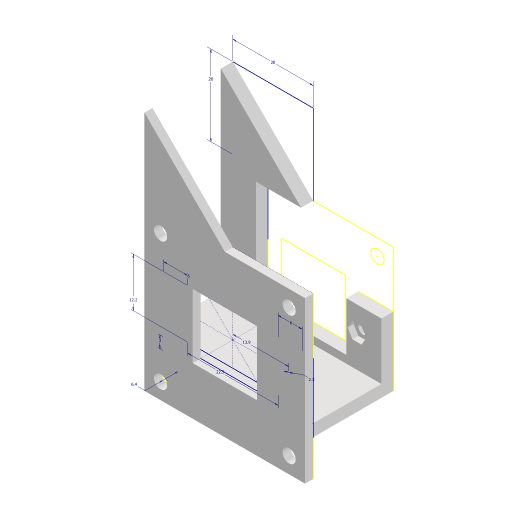
# Autodesk Inventor part: SG90_holder_1205
Saved by Autodesk Inventor 2024 (Build 280153000, 153)
## iProperties
Created: 2023-02-14
Part Number: SG90_holder_1205
Material: 一般
Document SubType Name: Modeling
Designer: USER
Density: 1 g/cm^3
Appearance: 預設
Author: USER
Autodesk Inventor part; units mm, degrees
ref_plane "YZ Plane" through (0, 0, 0) normal (1, 0, 0) x (0, 1, 0)
ref_plane "XZ Plane" through (0, 0, 0) normal (0, 1, 0) x (-1, 0, 0)
ref_plane "XY Plane" through (0, 0, 0) normal (0, 0, 1) x (1, 0, 0)
sketch "草圖11" plane through (0, 0, 0) normal (0, 0, 1) x (1, 0, 0)
  line L0 (0, 0) -> (22.5, 0)
  line L1 (22.5, 0) -> (22.5, -12.2)
  line L2 (22.5, -12.2) -> (0, -12.2)
  line L3 (0, -12.2) -> (0, 0)
  line L4 (-6, -18.2) -> (28.5, -18.2)
  line L5 (28.5, -18.2) -> (28.5, 6)
  line L6 (28.5, 6) -> (-6, 6)
  line L7 (-6, 6) -> (-6, -18.2)
  circle A0 centre (-2.65, -6.1) radius 1.15
  line L8 (0, -6.1) -> (22.5, -6.1) construction
  line L9 (11.25, 0) -> (11.25, -12.2) construction
  circle A1 centre (25.15, -6.1) radius 1.15
  line L10 (-6, 0) -> (0, 0) construction
  line L11 (22.5, 0) -> (28.5, 0) construction
  line L12 (-6, 0) -> (0, 0)
  line L13 (22.5, 0) -> (28.5, 0)
  line L14 (22.5, 0) -> (22.5, 6)
  line L15 (0, 0) -> (0, 6)
  dimension "d52" = 22.5
  dimension "d53" = 12.2
  dimension "d55" = 2.3
  dimension "d56" = 13.9
  dimension "d110" = 6
  constraints: 32 end point, 6 point on line, 5 equal length, 5 perpendicular, 4 midpoint, 2 centre point, 2 horizontal, 1 symmetric about line, 4 other
  measures "d52" distance of L1.end L2.end
  measures "d53" distance of L0.end L1.end
  measures "d55" diameter of A0
  measures "d56" distance from line of L9 A0.centre
  measures "d110" distance between parallel lines of L4 L2
extrude "擠出11" [suppressed]
sketch "草圖20" plane through (0, 0, 2) normal (0, 0, 1) x (1, 0, 0)
  line L0 (28.5, 0) -> (22.5, 0) projected
  line L1 (22.5, 0) -> (22.5, -12.2) projected
  line L2 (22.5, -12.2) -> (0, -12.2) projected
  line L3 (0, -12.2) -> (0, 0) projected
  line L4 (0, 0) -> (-6, 0) projected
  line L5 (-6, 0) -> (-6, -18.2) projected
  line L6 (-6, -18.2) -> (28.5, -18.2) projected
  line L7 (28.5, -18.2) -> (28.5, 0) projected
  circle A0 centre (-2.65, -6.1) radius 1.15 projected
  circle A1 centre (25.15, -6.1) radius 1.15 projected
  line L8 (-6, 0) -> (-4, 0)
  line L9 (-4, 0) -> (-4, -18.2)
  line L10 (-4, -18.2) -> (-6, -18.2)
  line L11 (-6, -18.2) -> (-6, 0)
  line L12 (-6, -18.2) -> (28.5, -18.2)
  line L13 (28.5, -18.2) -> (28.5, -16.2)
  line L14 (28.5, -16.2) -> (-6, -16.2)
  line L15 (-6, -16.2) -> (-6, -18.2)
  line L16 (-6, -18.2) -> (28.5, -18.2) projected
  point P0 (-4, -16.2)
  dimension "d97" = 2
  dimension "d98" = 2
  constraints: 16 end point, 4 parallel, 3 point on line, 2 horizontal, 2 perpendicular, 1 collinear
  measures "d97" distance between parallel lines of L5 L9
  measures "d98" distance between parallel lines of L6 L14
extrude "擠出17" [suppressed]
sketch "草圖21" plane through (0, 0, 22) normal (0, 0, 1) x (1, 0, 0)
  line L0 (-8.75, -26.1) -> (31.25, -26.1)
  line L1 (31.25, -26.1) -> (31.25, 13.9)
  line L2 (31.25, 13.9) -> (-8.75, 13.9)
  line L3 (-8.75, 13.9) -> (-8.75, -26.1)
  circle A0 centre (-2.65, -6.1) radius 1.15 projected
  line L4 (-8.75, -6.1) -> (31.25, -6.1) construction
  line L5 (11.25, -26.1) -> (11.25, 13.9) construction
  line L6 (28.5, -16.2) -> (-4, -16.2) construction
  line L7 (-4, -16.2) -> (-4, 0) construction
  line L8 (-4, 0) -> (-6, 0) construction
  line L9 (-6, 0) -> (-6, -18.2) construction
  line L10 (-6, -18.2) -> (28.5, -18.2) construction
  line L11 (28.5, -18.2) -> (28.5, -16.2) construction
  line L12 (-6, -18.2) -> (28.5, -18.2) construction
  line L13 (11.25, -18.2) -> (11.25, -16.2) construction
  line L14 (28.5, -16.2) -> (-4, -16.2) construction
  line L15 (1.25, 3.9) -> (21.25, 3.9)
  line L16 (21.25, 3.9) -> (21.25, -16.1)
  line L17 (21.25, -16.1) -> (1.25, -16.1)
  line L18 (1.25, -16.1) -> (1.25, 3.9)
  circle A1 centre (-4.75, -22.1) radius 3 construction
  circle A2 centre (-4.75, -22.1) radius 1.65
  circle A3 centre (-4.75, 9.9) radius 1.65
  circle A4 centre (27.25, -22.1) radius 1.65
  circle A5 centre (27.25, 9.9) radius 1.65
  line L19 (1.25, 3.9) -> (1.25, 13.9)
  line L20 (21.25, -16.1) -> (31.25, -16.1)
  point P0 (0, 0)
  dimension "d101" = 40
  dimension "d102" = 40
  dimension "d103" = 10
  dimension "d104" = 3.3
  dimension "d105" = 6
  dimension "d106" = 16
  dimension "d107" = 16
  constraints: 26 end point, 5 centre point, 5 midpoint, 5 perpendicular, 4 parallel, 4 point on line, 3 symmetric about line, 1 coincident, 1 collinear, 1 horizontal, 6 other
  measures "d101" distance of L1.end L2.end
  measures "d102" distance of L2.end L0.start
  measures "d103" distance between parallel lines of L2 L15
  measures "d104" diameter of A2
  measures "d105" diameter of A1
  measures "d106" distance from line of L4 A1.centre
  measures "d107" distance from line of L5 A1.centre
extrude "擠出18" [suppressed]
sketch "草圖22" plane through (0, 0, 0) normal (0, 0, 1) x (1, 0, 0)
  line L0 (-20, 20) -> (20, 20)
  line L1 (20, 20) -> (20, -20)
  line L2 (20, -20) -> (-20, -20)
  line L3 (-20, -20) -> (-20, 20)
  line L4 (0, -12.2) -> (0, 0) projected
  line L5 (-20, 20) -> (20, -20) construction
  line L6 (20, 20) -> (-20, -20) construction
  line L7 (-16, 16) -> (16, 16) construction
  line L8 (16, 16) -> (16, -16) construction
  line L9 (16, -16) -> (-16, -16) construction
  line L10 (-16, -16) -> (-16, 16) construction
  line L11 (-16, 16) -> (16, -16) construction
  line L12 (16, 16) -> (-16, -16) construction
  circle A0 centre (-16, 16) radius 1.65
  line L13 (20, 20) -> (-8, 20)
  line L14 (-8, 20) -> (-8, -8)
  line L15 (-8, -8) -> (20, -8)
  line L16 (20, -8) -> (20, 20)
  circle A1 centre (-16, -16) radius 1.65
  circle A2 centre (16, 16) radius 1.65
  circle A3 centre (16, -16) radius 1.65
  line L17 (-8, 8) -> (8, 8)
  line L18 (8, 8) -> (8, -8)
  line L19 (8, -8) -> (-8, -8)
  line L20 (-8, -8) -> (-8, 8)
  point P0 (20, -8)
  dimension "d118" = 40
  dimension "d119" = 16
  dimension "d120" = 3.3
  dimension "d121" = 12
  dimension "d124" = 32
  dimension "d127" = 32
  constraints: 40 end point, 8 parallel, 5 perpendicular, 4 centre point, 4 horizontal, 4 midpoint, 2 point on line, 1 coincident, 1 collinear, 1 vertical, 9 other
  measures "d118" distance of L0.start L0.end
  measures "d119" distance from line of L4.end L8
  measures "d120" diameter of A0
  measures "d121" distance between parallel lines of L2 L15
  measures "d124" distance of A0.centre A1.centre
  measures "d127" distance of A0.centre A2.centre
extrude "擠出19" add sketch "草圖22" along normal blind 2 contours L0 L14 L15 L1 L2 L3 | L0 L1 L15 L18 L17 L14
sketch "草圖23" plane through (0, 0, 0) normal (0, 0, -1) x (-1, 0, 0)
  line L0 (-11.25, 6.1) -> (11.25, 6.1)
  line L1 (11.25, 6.1) -> (11.25, -6.1)
  line L2 (11.25, -6.1) -> (-11.25, -6.1)
  line L3 (-11.25, -6.1) -> (-11.25, 6.1)
  circle A0 centre (-13.9, 0) radius 1.15
  line L4 (-11.25, 0) -> (11.25, 0) construction
  line L5 (0, 6.1) -> (0, -6.1) construction
  circle A1 centre (13.9, 0) radius 1.15
  line L6 (20, -20) -> (-20, -20) projected
  circle A2 centre (16, -16) radius 1.65 projected
  line L7 (20, 20) -> (-20, 20) construction
  line L8 (-20, 20) -> (-20, -20) construction
  line L9 (-20, -20) -> (20, -20) construction
  line L10 (20, -20) -> (20, 20) construction
  line L11 (20, 20) -> (-20, -20) construction
  line L12 (-20, 20) -> (20, -20) construction
  line L13 (17.25, 6.1) -> (-17.25, 6.1)
  line L14 (-17.25, 6.1) -> (-17.25, -11)
  line L15 (-17.25, -11) -> (17.25, -11)
  line L16 (17.25, -11) -> (17.25, 6.1)
  circle A3 centre (16, -16) radius 3.2 construction
  line L17 (17.25, -8) -> (-17.25, -8)
  line L18 (-8, -8) -> (8, -8) construction
  line L19 (20, 6.1) -> (17.25, 6.1)
  line L20 (17.25, -8) -> (20, -8)
  line L21 (17.25, -11) -> (20, -11)
  line L22 (20, 6.1) -> (20, -11)
  line L23 (20, 20) -> (20, -20) projected
  line L24 (-17.25, 6.1) -> (-20, 6.1)
  line L25 (-17.25, -8) -> (-20, -8)
  line L26 (-17.25, -11) -> (-20, -11)
  line L27 (-20, -11) -> (-20, 6.1)
  line L28 (-20, -20) -> (-20, 20) projected
  point P0 (0, 0)
  point P1 (0, 0)
  point P2 (0, 0)
  dimension "d132" = 22.5
  dimension "d134" = 2.3
  dimension "d135" = 13.9
  dimension "d162" = 12.2
  dimension "d163" = 6.4
  dimension "d164" = 6
  dimension "d165" = 6
  dimension "d166" = 3
  constraints: 50 end point, 8 midpoint, 8 perpendicular, 8 point on line, 7 parallel, 4 horizontal, 3 centre point, 3 collinear, 2 coincident, 1 symmetric about line, 1 other
  measures "d132" distance of L1.end L2.end
  measures "d134" diameter of A0
  measures "d135" distance from line of L5 A0.centre
  measures "d162" distance between parallel lines of L2 L0
  measures "d163" diameter of A3
  measures "d164" distance between parallel lines of L1 L16
  measures "d165" distance between parallel lines of L14 L3
  measures "d166" distance between parallel lines of L15 L17
extrude "擠出20" add sketch "草圖23" along normal blind 17 contours L17 L16 L15 L14 | L14 L26 L27 L25 | L20 L22 L21 L16
extrude "擠出21" add sketch "草圖23" along normal blind 3 from surface at 17 contours L3 L2 L1 L13 L16 L17 L14 | L14 L25 L27 L24 | L19 L22 L20 L16 | L17 L16 L15 L14 | L14 L26 L27 L25 | L20 L22 L21 L16
sketch "草圖25" plane through (-18.5, -8, -17) normal (0, 0, 1) x (1, 0, 0)
  line L0 (29.75, 14.1) -> (29.75, 1.9) projected
  line L1 (29.75, 1.9) -> (7.25, 1.9) projected
  line L2 (7.25, 1.9) -> (7.25, 14.1) projected
  circle A0 centre (32.4, 8) radius 1.15 projected
  circle A1 centre (4.6, 8) radius 1.15 projected
  line L3 (1.0097, 5.9187) -> (4.9457, 12.4467)
  line L4 (4.6073, 3.8501) -> (0.9219, 10.5227)
  line L5 (8.1976, 5.9314) -> (0.5762, 6.076)
  line L6 (8.1903, 10.0813) -> (4.2543, 3.5533)
  line L7 (4.5927, 12.1499) -> (8.2781, 5.4773)
  line L8 (1.0024, 10.0686) -> (8.6238, 9.924)
  line L9 (28.593, 10) -> (40.4698, 10)
  line L10 (28.7645, 5.7031) -> (34.7029, 15.9887)
  line L11 (32.5714, 3.7031) -> (26.633, 13.9887)
  line L12 (36.207, 6) -> (24.3302, 6)
  line L13 (36.0355, 10.2969) -> (30.0971, 0.0113)
  line L14 (32.2286, 12.2969) -> (38.167, 2.0113)
  line L15 (7.25, 14.1) -> (-1.5, 14.1) projected
  line L16 (-1.5, 14.1) -> (-1.5, 0) projected
  line L17 (-1.5, 0) -> (38.5, 0) projected
  line L18 (38.5, 0) -> (38.5, 14.1) projected
  line L19 (38.5, 14.1) -> (29.75, 14.1) projected
  point P0 (18.5, 8)
  point P1 (5.7924, 9.9777)
  point P2 (3.4835, 10.0216)
  point P3 (2.291, 8.0438)
  point P4 (3.4076, 6.0223)
  point P5 (5.7165, 5.9784)
  point P6 (6.909, 7.9562)
  point P7 (34.7094, 8)
  point P8 (33.5547, 10)
  point P9 (31.2453, 10)
  point P10 (30.0906, 8)
  point P11 (31.2453, 6)
  point P12 (33.5547, 6)
  dimension "d153" = 2
  dimension "d156" = 360
  dimension "d167" = 2
  dimension "d170" = 360
  constraints: 24 end point, 1 horizontal, 38 other
  measures "d153" distance from line of L3 A1.centre
  measures "d167" distance from line of L9 A0.centre
extrude "擠出22" cut sketch "草圖25" against normal blind 1.5 contours L9 L14 L13 L12 L11 L10 | L5 L4 L3 L8 L7 L6
sketch "草圖26" plane through (17.25, -11, -20) normal (0, 0, -1) x (-1, 0, 0)
  line L0 (6, 4.9) -> (28.5, 4.9) projected
  line L1 (6, 17.1) -> (6, 4.9) projected
  line L2 (37.25, 0) -> (-2.75, 0) projected
  line L3 (37.25, 17.1) -> (37.25, 0) projected
  line L4 (28.5, 17.1) -> (37.25, 17.1) projected
  line L5 (28.5, 4.9) -> (28.5, 17.1) projected
  circle A0 centre (3.35, 11) radius 1.15 projected
  circle A1 centre (31.15, 11) radius 1.15 projected
  line L6 (-2.75, 17.1) -> (6, 17.1) projected
  line L7 (-2.75, 0) -> (-2.75, 17.1) projected
  line L8 (37.25, 31) -> (37.25, 3) projected
  line L9 (-2.75, 31) -> (37.25, 31) projected
  line L10 (-2.75, 3) -> (-2.75, 31) projected
  line L11 (-2.75, 3) -> (9.25, 3) projected
  line L12 (9.25, 19) -> (9.25, 3) projected
  line L13 (25.25, 19) -> (9.25, 19) projected
  line L14 (25.25, 3) -> (25.25, 19) projected
  line L15 (25.25, 3) -> (37.25, 3) projected
  circle A2 centre (33.25, 27) radius 1.65 projected
  circle A3 centre (1.25, 27) radius 1.65 projected
  line L16 (37.25, 31) -> (28.5, 31)
  line L17 (28.5, 31) -> (28.5, 17.1)
  line L18 (28.5, 17.1) -> (37.25, 17.1)
  line L19 (37.25, 17.1) -> (37.25, 31)
  line L20 (37.25, 31) -> (37.25, 3) projected
  line L21 (37.25, 31) -> (17.25, 31)
  line L22 (17.25, 31) -> (17.25, 51)
  line L23 (17.25, 51) -> (37.25, 51)
  line L24 (37.25, 51) -> (37.25, 31)
  dimension "d190" = 20
  dimension "d191" = 20
  constraints: 16 end point, 4 parallel, 2 horizontal, 2 perpendicular
  measures "d190" distance of L22.end L23.end
  measures "d191" distance of L23.end L8.start
extrude "擠出23" add sketch "草圖26" against normal up to surface (3 mm away) contours L17 L9 L8 L4 | L22 L23 L24 L9 | A2
sketch "草圖27" plane through (0, 0, 2) normal (0, 0, 1) x (1, 0, 0)
  line L0 (-15.0924, -1.9777) -> (-16.209, 0.0438) projected
  line L1 (-16.209, 0.0438) -> (-15.0165, 2.0216) projected
  line L2 (-15.0165, 2.0216) -> (-12.7076, 1.9777) projected
  line L3 (-12.7076, 1.9777) -> (-11.591, -0.0438) projected
  line L4 (-11.591, -0.0438) -> (-12.7835, -2.0216) projected
  line L5 (-12.7835, -2.0216) -> (-15.0924, -1.9777) projected
  line L6 (11.5906, 0) -> (12.7453, 2) projected
  line L7 (12.7453, 2) -> (15.0547, 2) projected
  line L8 (15.0547, 2) -> (16.2094, 0) projected
  line L9 (16.2094, 0) -> (15.0547, -2) projected
  line L10 (15.0547, -2) -> (12.7453, -2) projected
  line L11 (12.7453, -2) -> (11.5906, 0) projected
  line L12 (11.25, 6.1) -> (11.25, -6.1) projected
  line L13 (11.25, -6.1) -> (-11.25, -6.1) projected
  line L14 (-11.25, -6.1) -> (-11.25, 20) projected
  line L15 (-20, 40) -> (-20, -8) projected
  line L16 (-20, -8) -> (20, -8) projected
  circle A0 centre (-16, -16) radius 1.65 projected
  circle A1 centre (16, -16) radius 1.65 projected
  line L17 (-20, 20) -> (-20, -20) projected
  line L18 (-20, -20) -> (20, -20) projected
  line L19 (20, -20) -> (20, 20) projected
  line L20 (8, -8) -> (-8, -8) projected
  line L21 (-8, -8) -> (-8, 8) projected
  line L22 (20, 20) -> (-20, 20) projected
  circle A2 centre (-16, 16) radius 1.65 projected
  line L23 (-8, 8) -> (8, 8) projected
  line L24 (8, 8) -> (8, -8) projected
  line L25 (20, -8) -> (20, 6.1) projected
  line L26 (20, 6.1) -> (11.25, 6.1) projected
  line L27 (-11.25, 20) -> (0, 20) projected
  line L28 (0, 20) -> (0, 40) projected
  line L29 (0, 40) -> (-20, 40) projected
  point P0 (0, 0)
  point P1 (-11.25, 20)
extrude "擠出24" [suppressed]
sketch "草圖30" plane through (0, 0, 2) normal (0, 0, 1) x (1, 0, 0)
  line L0 (-20, 40) -> (-20, -8) projected
  line L1 (-15.0924, -1.9777) -> (-16.209, 0.0438) projected
  line L2 (-16.209, 0.0438) -> (-15.0165, 2.0216) projected
  line L3 (-15.0165, 2.0216) -> (-12.7076, 1.9777) projected
  line L4 (-12.7076, 1.9777) -> (-11.591, -0.0438) projected
  line L5 (-11.591, -0.0438) -> (-12.7835, -2.0216) projected
  line L6 (-12.7835, -2.0216) -> (-15.0924, -1.9777) projected
  line L7 (11.5906, 0) -> (12.7453, 2) projected
  line L8 (12.7453, 2) -> (15.0547, 2) projected
  line L9 (15.0547, 2) -> (16.2094, 0) projected
  line L10 (16.2094, 0) -> (15.0547, -2) projected
  line L11 (15.0547, -2) -> (12.7453, -2) projected
  line L12 (12.7453, -2) -> (11.5906, 0) projected
  line L13 (-20, 40) -> (-20, -8) projected
  line L14 (-20, -8) -> (20, -8) projected
  line L15 (20, -8) -> (20, 6.1) projected
  line L16 (20, 6.1) -> (11.25, 6.1) projected
  line L17 (11.25, 6.1) -> (11.25, -6.1) projected
  line L18 (11.25, -6.1) -> (-11.25, -6.1) projected
  line L19 (-11.25, -6.1) -> (-11.25, 20) projected
  line L20 (-11.25, 20) -> (0, 20) projected
  line L21 (0, 20) -> (0, 40) projected
  line L22 (0, 40) -> (-20, 40) projected
  line L23 (20, 20) -> (-20, 20) projected
  line L24 (-11.25, 20) -> (-20, 20)
  point P0 (0, 0)
  constraints: 2 end point, 1 collinear
extrude "擠出27" add sketch "草圖30" against normal up to surface (2 mm away) contours L22 L21 L20 L23 L0
chamfer "倒角1" distance 20 angle 45 2 edges at (0, 40, 1) (0, 40, -18.5)
